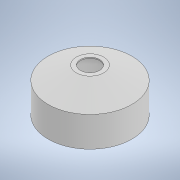
# Autodesk Inventor part: Parte superior
Saved by Autodesk Inventor 2022 (Build 260153000, 153)
## iProperties
Created: 2022-08-24
Part Number: Parte superior
Material: Generic
Document SubType Name: Modeling
Designer: Usuario
Density: 1 g/cm^3
Appearance: Default
Author: Usuario
Autodesk Inventor part; units mm, degrees
ref_plane "YZ Plane" through (0, 0, 0) normal (1, 0, 0) x (0, 1, 0)
ref_plane "XZ Plane" through (0, 0, 0) normal (0, 1, 0) x (-1, 0, 0)
ref_plane "XY Plane" through (0, 0, 0) normal (0, 0, 1) x (1, 0, 0)
sketch "Sketch1" plane through (0, 0, 0) normal (0, 1, 0) x (-1, 0, 0)
  line L0 (-12.75, 0) -> (-16.75, 0)
  line L1 (0, 12.75) -> (0, 16.75)
  line L2 (0, -12.75) -> (0, -16.75)
  line L3 (12.75, 0) -> (16.75, 0)
  arc A0 (-12.75, 0) -> (0, -12.75) centre (0, 0) ccw
  arc A1 (12.75, 0) -> (0, 12.75) centre (0, 0) ccw
  arc A2 (-16.75, 0) -> (0, -16.75) centre (0, 0) ccw
  arc A3 (16.75, 0) -> (0, 16.75) centre (0, 0) ccw
  constraints: 8 end point, 8 point on circle, 4 centre point, 3 point on line, 2 coincident, 1 horizontal, 1 perpendicular
extrude "Extrusion1" add sketch "Sketch1" along normal blind 3
sketch "Sketch2" plane through (0, 0, 0) normal (0, -1, 0) x (1, 0, 0)
  circle A0 centre (0, 0) radius 16.75
  arc A1 (0, -16.75) -> (16.75, 0) centre (0, 0) ccw projected
  circle A2 centre (0, 0) radius 20.75
  arc A3 (0, -16.75) -> (16.75, 0) centre (0, 0) ccw projected
  dimension "d4" = 4
  dimension "d5" = 33.5
  constraints: 2 centre point, 2 coincident
  measures "d4" radial gap between concentric circles of A2 A0
  measures "d5" diameter of A0
extrude "Extrusion2" add sketch "Sketch2" against normal blind 8
sketch "Sketch3" plane through (0, 0, 0) normal (1, 0, 0) x (0, 1, 0)
  line L0 (8, -20.75) -> (8, 20.75) projected
  line L1 (8, 16.75) -> (8, -16.75) projected
  line L2 (8, 16.75) -> (8, -16.75) projected
  line L3 (8, -16.75) -> (13, -16.75)
  line L4 (13, -16.75) -> (21, -6.75)
  line L5 (8, -20.75) -> (8, 20.75) projected
  line L6 (3, 0) -> (3, -12.75) projected
  line L7 (0, -12.75) -> (3, -12.75) projected
  line L8 (21, -6.75) -> (21, -4.75)
  line L9 (21.5, -4.75) -> (21.5, -6.8032)
  line L10 (14.9225, -20.75) -> (8, -20.75)
  line L11 (14.9225, -20.75) -> (21.5, -6.8032)
  line L12 (8, -16.75) -> (8, -20.75)
  line L13 (21, -4.75) -> (21.5, -4.75)
  line L14 (-4.3, 0) -> (25.8, 0) projected
  point P0 (0, 0)
  dimension "d8" = 5
  dimension "d9" = 8
  dimension "d10" = 6
  dimension "d11" = 2
  dimension "d12" = 0.5
  constraints: 16 end point, 1 collinear, 1 horizontal, 1 perpendicular, 1 vertical
  measures "d8" distance of L1.end L3.end
  measures "d9" horizontal distance of L4.end L3.end
  measures "d10" distance from line of L7 L4.end
  measures "d11" distance of L4.end L8.end
  measures "d12" distance between parallel lines of L8 L9
revolve "Revolution1" add sketch "Sketch3" angle 360 about axis through (0, -10, 0) along (0, 1, 0)
body "Solid1"
